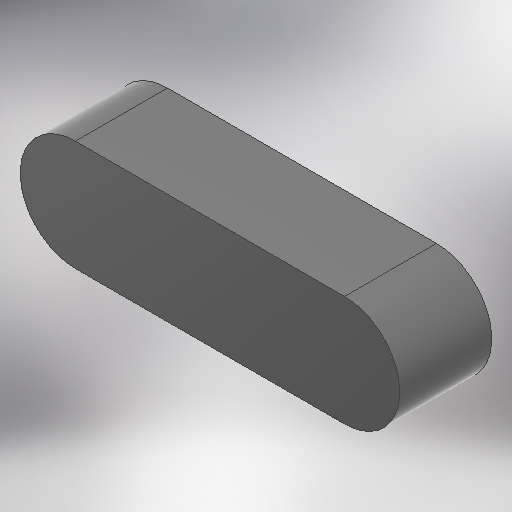
# Autodesk Inventor part: astra_camera
Saved by Autodesk Inventor 2026 (Build 300175050, 175E)
## iProperties
Created: 2025-07-05
Part Number: astra_camera
Material: Generic
Document SubType Name: Modeling
Designer: satom
Density: 1 g/cm^3
Appearance: Default
Author: satom
Autodesk Inventor part; units mm, degrees
ref_plane "YZ Plane" through (0, 0, 0) normal (1, 0, 0) x (0, 1, 0)
ref_plane "XZ Plane" through (0, 0, 0) normal (0, 1, 0) x (-1, 0, 0)
ref_plane "XY Plane" through (0, 0, 0) normal (0, 0, 1) x (1, 0, 0)
sketch "Sketch1" plane through (0, 0, 0) normal (0, 0, 1) x (1, 0, 0)
  line L0 (-58.5, 0) -> (58.5, 0) construction
  line L1 (-58.5, 24) -> (58.5, 24)
  line L2 (58.5, -24) -> (-58.5, -24)
  arc A0 (-58.5, 24) -> (-58.5, -24) centre (-58.5, 0) ccw
  arc A1 (58.5, -24) -> (58.5, 24) centre (58.5, 0) ccw
  point P0 (0, 0)
  dimension "d0" = 117
  dimension "d1" = 24
  constraints: 8 end point, 4 point on circle, 4 tangent, 2 centre point, 1 horizontal, 1 midpoint, 1 parallel
  measures "d0" distance of L1.start L1.end
  measures "d1" radius of A1
extrude "Extrusion1" add sketch "Sketch1" along normal blind 40
body "Solid1"
